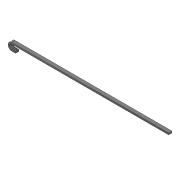
# Autodesk Inventor part: J15BF.1.30_Yaxis
Saved by Autodesk Inventor 2020 (Build 240168000, 168)
## iProperties
Created: 2020-06-16
Part Number: J15BF.1.30_Yaxis
Material: Generic
Document SubType Name: Modeling
Designer: hirohouse
Density: 1 g/cm^3
Appearance: Default
Author: hirohouse
Autodesk Inventor part; units mm, degrees
ref_plane "YZ Plane" through (0, 0, 0) normal (1, 0, 0) x (0, 1, 0)
ref_plane "XZ Plane" through (0, 0, 0) normal (0, 1, 0) x (-1, 0, 0)
ref_plane "XY Plane" through (0, 0, 0) normal (0, 0, 1) x (1, 0, 0)
sketch "Sketch1" plane through (0, 0, 0) normal (0, 0, 1) x (1, 0, 0)
  circle A0 centre (0, 0) radius 45
  line L0 (0, -45) -> (43, -45)
  line L1 (43, -45) -> (43, -25)
  line L2 (43, -25) -> (0, -25)
  line L3 (0, -25) -> (0, -45)
  line L4 (0, 45) -> (1850, 45)
  line L5 (1850, 45) -> (1850, 25)
  line L6 (1850, 25) -> (0, 25)
  line L7 (0, 25) -> (0, 45)
  circle A1 centre (0, 0) radius 25
  point P0 (0, -25)
  point P1 (0, 25)
  point P2 (13, -25)
  point P3 (-45, 0)
  dimension "d0" = 90
  dimension "d1" = 20
  dimension "d2" = 20
  dimension "d9" = 1850
  dimension "d10" = 58
  dimension "d11" = 30
  constraints: 16 end point, 4 parallel, 3 point on circle, 2 centre point, 2 coincident, 2 horizontal, 2 perpendicular, 2 point on line, 1 tangent, 1 vertical alignment
  measures "d0" diameter of A0
  measures "d1" distance of L4.end L5.end
  measures "d2" distance of L0.end L1.end
  measures "d9" distance of L4.start L4.end
  measures "d10" horizontal distance of point (13, -25) point (-45, 0)
  measures "d11" distance from line of L1 point (13, -25)
extrude "Extrusion1" add sketch "Sketch1" along normal blind 39 contours L7 A1 L3 A0 | L4 L5 L6 A0 | A0 L6 L7 | L3 L2 A0 | A0 L2 L1 L0
body "Solid1"
